Autodesk Inventor part; units mm, degrees
(part 2 of 2)
  line L255 (9.8203, 13.4042) -> (9.5423, 13.4042)
  line L256 (9.1736, 13.4042) -> (8.4447, 13.4042)
  spline S291 degree 2 poles (8.4447, 13.4042) (8.4589, 13.2453) (8.5071, 12.766) (8.5525, 12.6157) knots 0 0 0 1 2 2 2
  spline S292 degree 2 poles (8.5525, 12.6157) (8.6063, 12.4398) (8.8304, 12.2101) (9.029, 12.2101) knots 0 0 0 1 2 2 2
  spline S293 degree 2 poles (9.029, 12.2101) (9.2559, 12.2101) (9.4856, 12.4653) (9.4856, 12.7093) knots 0 0 0 1 2 2 2
  spline S294 degree 2 poles (9.4856, 12.7093) (9.4856, 12.9163) (9.3069, 13.2567) (9.1736, 13.4042) knots 0 0 0 1 2 2 2
  line L257 (7.6675, 15.8604) -> (7.6675, 15.8377)
  spline S295 degree 2 poles (7.6675, 15.8377) (7.6533, 15.7867) (7.6477, 15.676) (7.6477, 15.5995) knots 0 0 0 1 2 2 2
  spline S296 degree 2 poles (7.6477, 15.5995) (7.6477, 15.4208) (7.8037, 15.0691) (7.9568, 14.9102) knots 0 0 0 1 2 2 2
  line L258 (7.9568, 14.9102) -> (9.8203, 14.9102)
  line L259 (9.8203, 14.9102) -> (9.8203, 14.4678)
  line L260 (9.8203, 14.4678) -> (7.1939, 14.4678)
  line L261 (7.1939, 14.4678) -> (7.1939, 14.9102)
  line L262 (7.1939, 14.9102) -> (7.5853, 14.9102)
  spline S297 degree 2 poles (7.5853, 14.9102) (7.3697, 15.1513) (7.1939, 15.5115) (7.1939, 15.6817) knots 0 0 0 1 2 2 2
  spline S298 degree 2 poles (7.1939, 15.6817) (7.1939, 15.7498) (7.1995, 15.8179) (7.208, 15.8604) knots 0 0 0 1 2 2 2
  line L263 (7.208, 15.8604) -> (7.6675, 15.8604)
  constraints: 2 end point, 1 horizontal, 1 midpoint, 2 other
extrude "Extrusion2" cut sketch "Sketch3" against normal blind 1
body "Solid1"
